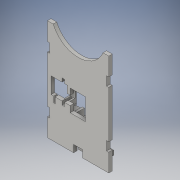
# Autodesk Inventor part: Backhalf
Saved by Autodesk Inventor 2016 (Build 200138000, 138)
## iProperties
Created: 2017-03-04
Part Number: Backhalf
Material: Generic
Document SubType Name: Modeling
Designer: Owner
Density: 1 g/cm^3
Appearance: Default
Author: Owner
Autodesk Inventor part; units mm, degrees
ref_plane "YZ Plane" through (0, 0, 0) normal (1, 0, 0) x (0, 1, 0)
ref_plane "XZ Plane" through (0, 0, 0) normal (0, 1, 0) x (-1, 0, 0)
ref_plane "XY Plane" through (0, 0, 0) normal (0, 0, 1) x (1, 0, 0)
sketch "Sketch1" plane through (0, 0, 0) normal (0, 0, 1) x (1, 0, 0)
  line L0 (31.75, -57.15) -> (31.75, 82.55)
  line L1 (31.75, 82.55) -> (-44.45, 82.55)
  line L2 (-44.45, 82.55) -> (-44.45, -57.15)
  arc A0 (-44.45, -57.15) -> (31.75, -57.15) centre (-6.35, -57.15) ccw
  line L3 (31.75, -57.15) -> (31.75, -209.55)
  line L4 (31.75, -209.55) -> (-44.45, -209.55)
  line L5 (-44.45, -209.55) -> (-44.45, -57.15)
  line L6 (31.75, -57.15) -> (-44.45, -57.15)
  circle A1 centre (-6.35, -57.15) radius 38.1
  point P0 (0, 0)
  dimension "d0" = 152.4
  dimension "d6" = 76.2
  constraints: 14 end point, 3 perpendicular, 2 centre point, 2 point on circle, 2 tangent, 1 coincident, 1 concentric, 1 vertical
  measures "d0" distance of L0.start L3.end
  measures "d6" distance of L3.end L4.end
extrude "Extrusion1" add sketch "Sketch1" against normal blind 5 contours L3 L4 L5 A0
sketch "Sketch2" plane through (0, 0, 0) normal (0, 0, 1) x (1, 0, 0)
  arc A0 (-44.45, -57.15) -> (31.75, -57.15) centre (-6.35, -57.15) ccw projected
  line L0 (31.75, -57.15) -> (31.75, -209.55) projected
  line L1 (-44.45, -57.15) -> (31.75, -57.15)
  line L2 (31.75, -57.15) -> (31.75, -72.15)
  line L3 (31.75, -72.15) -> (-44.45, -72.15)
  line L4 (-44.45, -72.15) -> (-44.45, -57.15)
  point P0 (0, 0)
  dimension "d3" = 15
  constraints: 8 end point, 2 parallel, 1 horizontal, 1 perpendicular, 1 point on line
  measures "d3" distance of L3.end L1.start
extrude "Extrusion2" cut sketch "Sketch2" against normal blind 5 contours L1 A0 L3 | A0 L3 L4 | L0 L3 A0
sketch "Sketch3" plane through (0, 0, -5) normal (0, 0, -1) x (-1, 0, 0)
  line L0 (16.51, -146.85) -> (16.51, -159.55) projected
  line L1 (-3.81, -159.55) -> (-3.81, -146.85) projected
  line L2 (16.51, -159.55) -> (16.51, -161.55)
  line L3 (-3.81, -146.85) -> (-3.81, -144.85)
  line L4 (4.857, -150.5555) -> (16.51, -161.55)
  line L5 (8.3369, -156.3105) -> (-3.81, -144.85)
  line L6 (16.51, -141.135) -> (12.446, -141.135)
  line L7 (16.51, -165.265) -> (12.446, -165.265)
  line L8 (16.51, -141.135) -> (17.51, -141.135)
  line L9 (17.51, -141.135) -> (17.51, -138.135)
  line L10 (17.51, -138.135) -> (-3.81, -138.135)
  line L11 (-3.81, -138.135) -> (-3.81, -163.265)
  line L12 (-3.81, -163.265) -> (-3.81, -164.265)
  line L13 (17.51, -138.135) -> (17.51, -165.265)
  line L14 (17.51, -165.265) -> (17.51, -168.265)
  line L15 (17.51, -168.265) -> (-3.81, -168.265)
  line L16 (-3.81, -168.265) -> (-3.81, -164.265)
  point P0 (0, 0)
  point P1 (17.51, -164.265)
  dimension "d7" = 2
  dimension "d8" = 2
  dimension "d28" = 1
  dimension "d29" = 3
  dimension "d30" = 1
  dimension "d73" = 3
  constraints: 30 end point, 5 perpendicular, 3 horizontal, 3 point on line, 3 vertical, 1 parallel, 4 other
  measures "d7" distance of L0.end L2.end
  measures "d8" distance of L1.end L3.end
  measures "d28" distance of L6.start L8.end
  measures "d29" distance of L8.end L9.end
  measures "d30" distance of L11.end L12.end
  measures "d73" distance of L13.end L14.end
extrude "Extrusion3" cut sketch "Sketch3" against normal blind 5
sketch "Sketch4" plane through (0, 0, -5) normal (0, 0, -1) x (-1, 0, 0)
  line L0 (-31.75, -72.15) -> (-28.673, -72.15) projected
  line L1 (-31.75, -72.15) -> (-36.75, -72.15)
  line L2 (-36.75, -72.15) -> (-36.75, -209.55)
  line L3 (-36.75, -209.55) -> (-36.75, -214.55)
  line L4 (-36.75, -214.55) -> (44.45, -214.55)
  line L5 (44.45, -214.55) -> (49.45, -214.55)
  line L6 (49.45, -214.55) -> (49.45, -72.15)
  line L7 (49.45, -72.15) -> (44.45, -72.15)
  line L8 (44.45, -72.15) -> (44.45, -214.55)
  line L9 (44.45, -214.55) -> (49.45, -214.55)
  line L10 (49.45, -214.55) -> (49.45, -72.15)
  line L11 (49.45, -214.55) -> (-36.75, -214.55)
  line L12 (-36.75, -214.55) -> (-36.75, -209.55)
  line L13 (-36.75, -209.55) -> (49.45, -209.55)
  line L14 (49.45, -209.55) -> (49.45, -214.55)
  line L15 (-36.75, -214.55) -> (-31.75, -214.55)
  line L16 (-31.75, -214.55) -> (-31.75, -72.15)
  line L17 (-31.75, -72.15) -> (-36.75, -72.15)
  line L18 (-36.75, -72.15) -> (-36.75, -214.55)
  point P0 (0, 0)
  dimension "d11" = 5
  dimension "d12" = 5
  dimension "d13" = 5
  constraints: 36 end point, 6 parallel, 6 perpendicular, 4 horizontal, 3 point on line
  measures "d11" distance of L0.start L1.end
  measures "d12" distance of L2.end L3.end
  measures "d13" distance of L4.end L5.end
extrude "Extrusion4" add sketch "Sketch4" against normal blind 5
sketch "Sketch6" plane through (-49.45, -214.55, 0) normal (0, -1, 0) x (1, 0, 0)
  line L0 (32.94, 0) -> (53.26, 0) projected
  line L1 (43.1, 0) -> (36.75, 0)
  line L2 (36.75, 0) -> (49.45, 0)
  line L3 (86.2, -5) -> (0, -5) projected
  line L4 (49.45, 0) -> (36.75, 0)
  line L5 (36.75, 0) -> (36.75, -5)
  line L6 (36.75, -5) -> (49.45, -5)
  line L7 (49.45, -5) -> (49.45, 0)
  point P0 (64.1616, -5)
  dimension "d18" = 6.35
  dimension "d19" = 12.7
  constraints: 12 end point, 2 parallel, 2 point on line, 1 collinear, 1 horizontal, 1 midpoint, 1 perpendicular
  measures "d18" distance of L1.start L1.end
  measures "d19" distance of L1.end L2.end
extrude "Extrusion6" add sketch "Sketch6" along normal blind 10.16
sketch "Sketch7" plane through (0, 0, -5) normal (0, 0, -1) x (-1, 0, 0)
  line L0 (12.7, -224.71) -> (0, -224.71) projected
  line L1 (6.35, -224.71) -> (6.35, -220.9)
  circle A0 centre (6.35, -220.9) radius 1.75
  point P0 (0, 0)
  dimension "d26" = 3.81
  dimension "d27" = 3.5
  constraints: 2 end point, 1 centre point, 1 coincident, 1 midpoint, 1 vertical
  measures "d26" distance of L1.start L1.end
  measures "d27" diameter of A0
extrude "Extrusion7" cut sketch "Sketch7" against normal blind 6.35
sketch "Sketch8" plane through (0, 0, -5) normal (0, 0, -1) x (-1, 0, 0)
  line L0 (44.45, -136.69) -> (28.448, -136.69) projected
  line L1 (44.45, -158.28) -> (44.45, -137.96) projected
  line L2 (44.45, -136.69) -> (44.45, -137.96) projected
  line L3 (44.45, -158.28) -> (44.45, -159.55) projected
  line L4 (44.45, -159.55) -> (28.448, -159.55) projected
  line L5 (39.116, -159.55) -> (40.132, -159.55) projected
  line L6 (39.116, -159.55) -> (39.116, -162.09) projected
  line L7 (40.132, -162.09) -> (39.116, -162.09) projected
  line L8 (40.132, -159.55) -> (40.132, -162.09) projected
  line L9 (25.908, -137.96) -> (21.59, -137.96) projected
  line L10 (21.59, -153.2) -> (21.59, -137.96) projected
  line L11 (21.59, -158.28) -> (21.59, -153.2) projected
  line L12 (25.908, -158.28) -> (21.59, -158.28) projected
  line L13 (25.908, -158.28) -> (25.908, -164.122) projected
  line L14 (25.908, -164.122) -> (28.448, -164.122) projected
  line L15 (28.448, -158.28) -> (28.448, -164.122) projected
  line L16 (44.45, -158.28) -> (28.448, -158.28) projected
  line L17 (44.45, -158.28) -> (44.45, -137.96) projected
  line L18 (44.45, -137.96) -> (28.448, -137.96) projected
  line L19 (28.448, -132.118) -> (28.448, -137.96) projected
  line L20 (25.908, -132.118) -> (28.448, -132.118) projected
  line L21 (25.908, -132.118) -> (25.908, -137.96) projected
  line L22 (25.908, -136.69) -> (21.59, -136.69) projected
  line L23 (21.59, -136.69) -> (21.59, -137.96) projected
  line L24 (25.908, -159.55) -> (21.59, -159.55) projected
  line L25 (21.59, -159.55) -> (16.51, -159.55)
  line L26 (21.59, -146.85) -> (16.51, -146.85)
  line L27 (17.51, -140.135) -> (17.51, -166.265) projected
  line L28 (44.45, -159.55) -> (21.59, -159.55)
  line L29 (21.59, -159.55) -> (21.59, -136.69)
  line L30 (21.59, -136.69) -> (44.45, -136.69)
  line L31 (44.45, -136.69) -> (44.45, -159.55)
  line L32 (28.448, -132.118) -> (25.908, -132.118)
  line L33 (25.908, -132.118) -> (25.908, -136.69)
  line L34 (25.908, -136.69) -> (28.448, -136.69)
  line L35 (28.448, -136.69) -> (28.448, -132.118)
  line L36 (25.908, -159.55) -> (28.448, -159.55)
  line L37 (28.448, -159.55) -> (28.448, -164.122)
  line L38 (28.448, -164.122) -> (25.908, -164.122)
  line L39 (25.908, -164.122) -> (25.908, -159.55)
  line L40 (40.132, -162.09) -> (39.116, -162.09)
  line L41 (39.116, -162.09) -> (39.116, -159.55)
  line L42 (39.116, -159.55) -> (40.132, -159.55)
  line L43 (40.132, -159.55) -> (40.132, -162.09)
  line L44 (16.51, -146.85) -> (21.59, -146.85)
  line L45 (21.59, -146.85) -> (21.59, -159.55)
  line L46 (21.59, -159.55) -> (16.51, -159.55)
  line L47 (16.51, -159.55) -> (16.51, -146.85)
  line L48 (40.132, -159.55) -> (40.64, -159.55)
  line L49 (40.64, -159.55) -> (40.64, -167.805)
  line L50 (40.64, -167.805) -> (39.116, -167.805)
  line L51 (39.116, -167.805) -> (38.608, -167.805)
  line L52 (38.608, -167.805) -> (38.608, -159.55)
  line L53 (40.64, -167.805) -> (38.608, -167.805)
  line L54 (38.608, -167.805) -> (38.608, -159.55)
  line L55 (38.608, -159.55) -> (40.64, -159.55)
  line L56 (40.64, -159.55) -> (40.64, -167.805)
  line L57 (28.448, -136.69) -> (28.948, -136.69)
  line L58 (28.948, -136.69) -> (28.948, -132.118)
  line L59 (28.948, -132.118) -> (28.948, -131.618)
  line L60 (28.948, -131.618) -> (25.908, -131.618)
  line L61 (25.908, -131.618) -> (25.408, -131.618)
  line L62 (25.408, -131.618) -> (25.408, -136.69)
  line L63 (44.45, -148.12) -> (42.0007, -148.12)
  line L64 (28.448, -164.122) -> (28.448, -158.28)
  line L65 (25.908, -164.122) -> (28.448, -164.122)
  line L66 (25.908, -164.122) -> (25.908, -158.28)
  line L67 (28.448, -164.122) -> (25.908, -164.122)
  line L68 (25.908, -164.122) -> (25.908, -159.55)
  line L69 (28.448, -159.55) -> (28.448, -164.122)
  line L70 (28.948, -159.55) -> (28.948, -164.122)
  line L71 (28.948, -164.122) -> (28.948, -164.622)
  line L72 (28.948, -164.622) -> (25.908, -164.622)
  line L73 (25.908, -164.622) -> (25.408, -164.622)
  line L74 (25.408, -164.622) -> (25.408, -159.55)
  line L75 (28.948, -159.55) -> (25.408, -159.55)
  line L76 (25.408, -159.55) -> (25.408, -164.622)
  line L77 (25.408, -164.622) -> (28.948, -164.622)
  line L78 (28.948, -164.622) -> (28.948, -159.55)
  point P0 (0, 0)
  dimension "d33" = 0.508
  dimension "d34" = 8.255
  dimension "d35" = 0.508
  dimension "d45" = 0.5
  dimension "d46" = 0.5
  dimension "d47" = 0.5
  constraints: 100 end point, 14 parallel, 12 perpendicular, 10 horizontal, 9 point on line, 9 symmetric about line, 1 midpoint, 1 vertical, 3 other
  measures "d33" distance of L42.end L48.end
  measures "d34" distance of L48.end L49.end
  measures "d35" distance of L50.end L51.end
  measures "d45" distance of L34.end L57.end
  measures "d46" distance of L58.end L59.end
  measures "d47" distance of L60.end L61.end
extrude "Extrusion8" cut sketch "Sketch8" against normal blind 25.4
sketch "Sketch9" plane through (0, 0, -5) normal (0, 0, -1) x (-1, 0, 0)
  line L0 (25.908, -132.118) -> (28.448, -132.118) projected
  line L1 (28.448, -132.118) -> (28.948, -132.118)
  line L2 (28.948, -132.118) -> (28.948, -131.618)
  line L3 (28.948, -131.618) -> (30.948, -131.618)
  line L4 (30.948, -131.618) -> (30.948, -136.69)
  line L5 (44.45, -136.69) -> (28.948, -136.69) projected
  line L6 (30.948, -136.69) -> (30.948, -136.19)
  line L7 (30.948, -136.19) -> (28.948, -136.19)
  line L8 (28.948, -136.19) -> (28.948, -131.618)
  line L9 (30.948, -131.618) -> (30.948, -129.618)
  line L10 (30.948, -129.618) -> (25.908, -129.618)
  line L11 (27.178, -132.118) -> (27.178, -133.3917)
  line L12 (28.448, -132.118) -> (25.908, -132.118)
  line L13 (25.908, -132.118) -> (25.408, -132.118)
  line L14 (25.408, -132.118) -> (25.408, -131.618)
  line L15 (25.408, -131.618) -> (23.408, -131.618)
  line L16 (23.408, -131.618) -> (23.408, -136.69)
  line L17 (9.906, -136.69) -> (25.908, -136.69)
  line L18 (23.408, -136.69) -> (23.408, -136.19)
  line L19 (23.408, -136.19) -> (25.408, -136.19)
  line L20 (25.408, -136.19) -> (25.408, -131.618)
  line L21 (23.408, -131.618) -> (23.408, -129.618)
  line L22 (23.408, -129.618) -> (28.448, -129.618)
  line L23 (28.948, -131.618) -> (25.408, -131.618)
  line L24 (44.45, -159.55) -> (44.45, -136.69) projected
  line L25 (44.45, -148.12) -> (41.4953, -148.12)
  line L26 (25.908, -164.122) -> (28.448, -164.122)
  line L27 (28.448, -164.122) -> (28.948, -164.122)
  line L28 (28.948, -164.122) -> (28.948, -164.622)
  line L29 (28.948, -164.622) -> (30.948, -164.622)
  line L30 (30.948, -164.622) -> (30.948, -159.55)
  line L31 (44.45, -159.55) -> (28.448, -159.55)
  line L32 (30.948, -159.55) -> (30.948, -160.05)
  line L33 (30.948, -160.05) -> (28.948, -160.05)
  line L34 (28.948, -160.05) -> (28.948, -164.622)
  line L35 (30.948, -164.622) -> (30.948, -166.622)
  line L36 (30.948, -166.622) -> (25.908, -166.622)
  line L37 (27.178, -164.122) -> (27.178, -162.8483)
  line L38 (28.448, -164.122) -> (25.908, -164.122)
  line L39 (25.908, -164.122) -> (25.408, -164.122)
  line L40 (25.408, -164.122) -> (25.408, -164.622)
  line L41 (25.408, -164.622) -> (23.408, -164.622)
  line L42 (23.408, -164.622) -> (23.408, -159.55)
  line L43 (9.906, -159.55) -> (25.908, -159.55)
  line L44 (23.408, -159.55) -> (23.408, -160.05)
  line L45 (23.408, -160.05) -> (25.408, -160.05)
  line L46 (25.408, -160.05) -> (25.408, -164.622)
  line L47 (23.408, -164.622) -> (23.408, -166.622)
  line L48 (23.408, -166.622) -> (28.448, -166.622)
  line L49 (28.948, -164.622) -> (25.408, -164.622)
  line L50 (23.408, -131.618) -> (30.948, -131.618)
  line L51 (30.948, -131.618) -> (30.948, -129.618)
  line L52 (30.948, -129.618) -> (23.408, -129.618)
  line L53 (23.408, -129.618) -> (23.408, -131.618)
  line L54 (30.948, -166.622) -> (23.408, -166.622)
  line L55 (23.408, -166.622) -> (23.408, -164.622)
  line L56 (23.408, -164.622) -> (30.948, -164.622)
  line L57 (30.948, -164.622) -> (30.948, -166.622)
  line L58 (28.948, -136.19) -> (30.948, -136.19)
  line L59 (30.948, -136.19) -> (30.948, -131.618)
  line L60 (30.948, -131.618) -> (28.948, -131.618)
  line L61 (28.948, -131.618) -> (28.948, -136.19)
  line L62 (25.408, -136.19) -> (23.408, -136.19)
  line L63 (23.408, -136.19) -> (23.408, -131.618)
  line L64 (23.408, -131.618) -> (25.408, -131.618)
  line L65 (25.408, -131.618) -> (25.408, -136.19)
  line L66 (28.948, -164.622) -> (30.948, -164.622)
  line L67 (30.948, -164.622) -> (30.948, -160.05)
  line L68 (30.948, -160.05) -> (28.948, -160.05)
  line L69 (28.948, -160.05) -> (28.948, -164.622)
  line L70 (25.408, -164.622) -> (23.408, -164.622)
  line L71 (23.408, -164.622) -> (23.408, -160.05)
  line L72 (23.408, -160.05) -> (25.408, -160.05)
  line L73 (25.408, -160.05) -> (25.408, -164.622)
  point P0 (0, 0)
  point P1 (28.448, -136.69)
  dimension "d36" = 0.5
  dimension "d37" = 0.5
  dimension "d38" = 2
  dimension "d39" = 0.5
  dimension "d40" = 2
  constraints: 142 end point, 37 symmetric about line, 12 parallel, 12 point on line, 10 horizontal, 10 perpendicular, 2 midpoint, 1 collinear, 1 vertical
  measures "d36" distance of L0.end L1.end
  measures "d37" distance of L1.end L2.end
  measures "d38" distance of L2.end L3.end
  measures "d39" distance of L4.end L6.end
  measures "d40" distance of L3.end L9.end
extrude "Extrusion9" add sketch "Sketch9" along normal blind 7.6962 contours L20 L19 L16 L15 L14 | L15 L21 L22 L10 L9 L3 L23 | L2 L3 L4 L7 L8 | L40 L41 L42 L45 L46 | L49 L29 L35 L36 L48 L47 L41 | L34 L33 L30 L29 L28
sketch "Sketch10" plane through (0, 0, -12.6962) normal (0, 0, -1) x (-1, 0, 0)
  line L0 (30.948, -129.618) -> (30.948, -136.19) projected
  line L1 (23.408, -160.05) -> (23.408, -166.622) projected
  line L2 (30.948, -129.618) -> (23.408, -129.618)
  line L3 (23.408, -129.618) -> (23.408, -166.622)
  line L4 (23.408, -166.622) -> (30.948, -166.622)
  line L5 (30.948, -166.622) -> (30.948, -129.618)
  point P0 (0, 0)
  constraints: 8 end point, 2 parallel, 1 horizontal, 1 perpendicular
extrude "Extrusion10" add sketch "Sketch10" along normal blind 2.0066
ref_plane "Work Plane1" through (-5.588, -193.548, -26.4528) normal (1, 0, 0) x (0, 0, 1)
sketch "Sketch11" plane through (-5.588, -193.548, -26.4528) normal (1, 0, 0) x (0, 0, 1)
  line L0 (6.35, -16.002) -> (6.35, -10.16) projected
  line L1 (6.35, -16.002) -> (6.35, -18.502)
  line L2 (6.35, 10.16) -> (6.35, 16.002) projected
  line L3 (6.35, 16.002) -> (6.35, 18.502)
  line L4 (21.4528, -121.398) -> (21.4528, 21.002) projected
  line L5 (6.35, -18.502) -> (21.4528, -18.502)
  line L6 (21.4528, -18.502) -> (21.4528, 18.502)
  line L7 (21.4528, 18.502) -> (6.35, 18.502)
  line L8 (6.35, 18.502) -> (6.35, -18.502)
  point P0 (26.4528, -193.548)
  dimension "d48" = 2.5
  dimension "d49" = 2.5
  constraints: 12 end point, 2 parallel, 2 vertical, 1 horizontal, 1 perpendicular, 1 point on line
  measures "d48" distance of L0.start L1.end
  measures "d49" distance of L2.end L3.end
extrude "Extrusion11" add sketch "Sketch11" against normal blind 5.04
sketch "Sketch12" plane through (-5.588, -193.548, -26.4528) normal (1, 0, 0) x (0, 0, -1)
  line L0 (-6.35, 18.502) -> (-21.4528, 18.502) projected
  line L1 (-21.4528, -18.502) -> (-21.4528, 18.502) projected
  line L2 (-21.4528, -18.502) -> (-6.35, -18.502) projected
  line L3 (-6.35, -18.502) -> (-6.35, 18.502) projected
  point P0 (-26.4528, 193.548)
extrude "Extrusion12" add sketch "Sketch12" along normal blind 10
sketch "Sketch13" plane through (-10.628, -212.05, -20.1028) normal (0, 0, -1) x (-1, 0, 0)
  line L0 (-21.042, 28.662) -> (-5.04, 28.662) projected
  line L1 (-21.042, 28.662) -> (-21.042, 8.342) projected
  line L2 (-21.042, 8.342) -> (-5.04, 8.342) projected
  line L3 (-5.04, 2.5) -> (-5.04, 8.342) projected
  line L4 (-2.5, 2.5) -> (-5.04, 2.5) projected
  line L5 (-2.5, 2.5) -> (-2.5, 8.342) projected
  line L6 (-2.5, 8.342) -> (1.818, 8.342) projected
  line L7 (1.818, 13.422) -> (1.818, 8.342) projected
  line L8 (1.818, 28.662) -> (1.818, 13.422) projected
  line L9 (-2.5, 28.662) -> (1.818, 28.662) projected
  line L10 (-2.5, 28.662) -> (-2.5, 34.504) projected
  line L11 (-2.5, 34.504) -> (-5.04, 34.504) projected
  line L12 (-5.04, 28.662) -> (-5.04, 34.504) projected
  line L13 (-2.5, 29.932) -> (1.818, 29.932) projected
  line L14 (-21.042, 29.932) -> (-5.04, 29.932) projected
  line L15 (-2.5, 7.072) -> (1.818, 7.072) projected
  line L16 (-21.042, 7.072) -> (-5.04, 7.072) projected
  line L17 (-2.5, 29.932) -> (-2, 29.932)
  line L18 (-2, 29.932) -> (-2, 30.432)
  line L19 (-2, 30.432) -> (0, 30.432)
  line L20 (0, 37.004) -> (0, 0) projected
  line L21 (-2, 30.432) -> (-2, 34.504)
  line L22 (-2, 34.504) -> (-2, 35.004)
  line L23 (-2, 35.004) -> (-5.04, 35.004)
  line L24 (-5.04, 35.004) -> (-5.54, 35.004)
  line L25 (-5.54, 35.004) -> (-5.54, 29.932)
  line L26 (-5.54, 29.932) -> (-7.54, 29.932)
  line L27 (-7.54, 29.932) -> (-7.54, 35.004)
  line L28 (-7.54, 35.004) -> (-7.54, 37.004)
  line L29 (-15.04, 37.004) -> (0, 37.004) projected
  line L30 (-7.54, 37.004) -> (0, 37.004)
  line L31 (0, 37.004) -> (0, 30.432)
  line L32 (-2, 29.932) -> (0, 29.932)
  line L33 (0, 29.932) -> (0, 37.004)
  line L34 (0, 37.004) -> (-2, 37.004)
  line L35 (-2, 37.004) -> (-2, 29.932)
  line L36 (-21.042, 18.502) -> (-17.938, 18.502)
  line L37 (-21.042, 8.342) -> (-5.04, 8.342)
  line L38 (1.818, 8.342) -> (1.818, 23.582)
  line L39 (-2.5, 8.342) -> (1.818, 8.342)
  line L40 (-2.5, 8.342) -> (-2.5, 2.5)
  line L41 (-2.5, 2.5) -> (-5.04, 2.5)
  line L42 (-5.04, 8.342) -> (-5.04, 2.5)
  line L43 (-2.5, 7.072) -> (1.818, 7.072)
  line L44 (-21.042, 7.072) -> (-5.04, 7.072)
  line L45 (-2.5, 7.072) -> (-2, 7.072)
  line L46 (-2, 7.072) -> (-2, 6.572)
  line L47 (-2, 6.572) -> (0, 6.572)
  line L48 (0, 0) -> (0, 37.004)
  line L49 (-2, 6.572) -> (-2, 2.5)
  line L50 (-2, 2.5) -> (-2, 2)
  line L51 (-2, 2) -> (-5.04, 2)
  line L52 (-5.04, 2) -> (-5.54, 2)
  line L53 (-5.54, 2) -> (-5.54, 7.072)
  line L54 (-5.54, 7.072) -> (-7.54, 7.072)
  line L55 (-7.54, 7.072) -> (-7.54, 2)
  line L56 (-7.54, 2) -> (-7.54, 0)
  line L57 (-15.04, 0) -> (0, 0)
  line L58 (-7.54, 0) -> (0, 0)
  line L59 (0, 0) -> (0, 6.572)
  line L60 (-2, 7.072) -> (0, 7.072)
  line L61 (0, 7.072) -> (0, 0)
  line L62 (0, 0) -> (-2, 0)
  line L63 (-2, 0) -> (-2, 7.072)
  point P0 (-10.628, 212.05)
  dimension "d0" = 152.4
  dimension "d19" = 12.7
  dimension "d28" = 1
  dimension "d29" = 3
  dimension "d30" = 1
  dimension "d73" = 3
  dimension "d54" = 0.5
  dimension "d55" = 0.5
  dimension "d56" = 2
  dimension "d57" = 0.5
  dimension "d58" = 0.5
  dimension "d59" = 2
  dimension "d60" = 2
  constraints: 74 end point, 17 symmetric about line, 16 point on line, 4 perpendicular, 3 parallel, 2 horizontal, 1 collinear, 1 midpoint, 1 vertical
  measures "d54" distance of L13.start L17.end
  measures "d55" distance of L17.end L18.end
  measures "d56" distance of L18.end L19.end
  measures "d57" distance of L21.end L22.end
  measures "d58" distance of L23.end L24.end
  measures "d59" distance of L25.end L26.end
  measures "d60" distance of L27.end L28.end
extrude "Extrusion13" add sketch "Sketch13" along normal blind 12 contours L14 L27 L28 L29 L35 L23 L24 L25 | L53 L52 L51 L63 L57 L56 L55 L16 | L35 L29 L20 L19 L21 L22 | L15 L20 L47 L46 | L50 L49 L47 L20 L57 L63
sketch "Sketch14" plane through (-30.948, -166.622, -5) normal (-1, 0, 0) x (0, 0, 1)
  line L0 (-9.7028, 18.744) -> (-9.7028, -2.006) projected
  line L1 (0, 94.472) -> (0, -47.928) projected
  line L2 (-9.7028, 0) -> (0, 0)
  line L3 (0, 0) -> (0, -2.006)
  line L4 (0, -2.006) -> (-9.7028, -2.006)
  line L5 (-9.7028, -2.006) -> (-9.7028, 0)
  point P0 (5, 166.622)
  constraints: 8 end point, 2 parallel, 1 horizontal, 1 perpendicular, 1 point on line
extrude "Extrusion14" add sketch "Sketch14" against normal blind 7.5438
sketch "Sketch15" plane through (0, 0, -5) normal (0, 0, -1) x (-1, 0, 0)
  line L0 (36.09, -168.628) -> (36.09, -191.4473) projected
  line L1 (36.09, -168.628) -> (36.09, -191.4473) projected
  line L2 (21.59, -168.628) -> (21.59, -191.4473) projected
  line L3 (36.09, -191.4473) -> (36.09, -186.4473)
  line L4 (36.09, -168.628) -> (36.09, -173.628)
  line L5 (36.09, -186.4473) -> (39.09, -186.4473)
  line L6 (39.09, -186.4473) -> (39.09, -173.628)
  line L7 (39.09, -173.628) -> (36.09, -173.628)
  line L8 (36.09, -173.628) -> (36.09, -186.4473)
  line L9 (21.59, -168.628) -> (21.59, -173.628)
  line L10 (21.59, -173.628) -> (18.59, -173.628)
  line L11 (18.59, -173.628) -> (18.59, -186.4473)
  line L12 (18.59, -186.4473) -> (21.59, -186.4473)
  line L13 (21.59, -186.4473) -> (21.59, -173.628)
  point P0 (0, 0)
  dimension "d65" = 5
  dimension "d66" = 5
  dimension "d67" = 3
  dimension "d68" = 3
  constraints: 22 end point, 4 parallel, 3 point on line, 2 horizontal, 2 perpendicular
  measures "d65" distance of L0.end L3.end
  measures "d66" distance of L0.start L4.end
  measures "d67" distance of L6.end L7.end
  measures "d68" distance of L9.end L10.end
extrude "Extrusion15" add sketch "Sketch15" along normal blind 16
sketch "Sketch16" plane through (-39.09, -186.4473, -5) normal (0, -1, 0) x (1, 0, 0)
  line L0 (3, -13.4528) -> (17.5, -13.4528) projected
  line L1 (0, 0) -> (0, -16) projected
  line L2 (0, -13.4528) -> (20.5, -13.4528)
  line L3 (20.5, -13.4528) -> (20.5, 0)
  line L4 (20.5, 0) -> (0, 0)
  line L5 (0, 0) -> (0, -13.4528)
  point P0 (39.09, 5)
  constraints: 8 end point, 2 parallel, 1 horizontal, 1 perpendicular, 1 point on line
extrude "Extrusion16" add sketch "Sketch16" against normal blind 12.819
sketch "Sketch17" plane through (0, 0, -5) normal (0, 0, -1) x (-1, 0, 0)
  line L0 (-7.25, -200.427) -> (-26.75, -200.427) projected
  line L1 (-26.75, -200.427) -> (-26.75, -202.177) projected
  line L2 (-7.25, -202.177) -> (-26.75, -202.177) projected
  line L3 (-7.25, -200.427) -> (-7.25, -202.177) projected
  line L4 (-7.25, -200.427) -> (-11.25, -200.427)
  line L5 (-11.25, -200.427) -> (-11.25, -200.177)
  line L6 (-11.25, -200.177) -> (-11.25, -198.177)
  line L7 (-11.25, -198.177) -> (-7.25, -198.177)
  line L8 (-7.25, -198.177) -> (-5.25, -198.177)
  line L9 (-11.25, -200.177) -> (-7.25, -200.177)
  line L10 (-7.25, -200.177) -> (-7, -200.177)
  line L11 (-7, -200.177) -> (-7, -202.177)
  line L12 (-7, -202.177) -> (-7, -202.427)
  line L13 (-7, -202.427) -> (-11.25, -202.427)
  line L14 (-11.25, -202.427) -> (-11.25, -204.427)
  line L15 (-11.25, -204.427) -> (-5.25, -204.427)
  line L16 (-5.25, -204.427) -> (-5.25, -198.177)
  line L17 (-17, -202.177) -> (-17, -205.7109)
  line L18 (-26.75, -200.427) -> (-7.25, -200.427)
  line L19 (-26.75, -202.177) -> (-7.25, -202.177)
  line L20 (-26.75, -200.427) -> (-26.75, -202.177)
  line L21 (-26.75, -200.427) -> (-22.75, -200.427)
  line L22 (-22.75, -200.427) -> (-22.75, -200.177)
  line L23 (-22.75, -200.177) -> (-22.75, -198.177)
  line L24 (-22.75, -198.177) -> (-26.75, -198.177)
  line L25 (-26.75, -198.177) -> (-28.75, -198.177)
  line L26 (-22.75, -200.177) -> (-26.75, -200.177)
  line L27 (-26.75, -200.177) -> (-27, -200.177)
  line L28 (-27, -200.177) -> (-27, -202.177)
  line L29 (-27, -202.177) -> (-27, -202.427)
  line L30 (-27, -202.427) -> (-22.75, -202.427)
  line L31 (-22.75, -202.427) -> (-22.75, -204.427)
  line L32 (-22.75, -204.427) -> (-28.75, -204.427)
  line L33 (-28.75, -204.427) -> (-28.75, -198.177)
  point P0 (0, 0)
  dimension "d74" = 4
  dimension "d75" = 0.25
  dimension "d76" = 2
  dimension "d77" = 2
  dimension "d78" = 0.25
  dimension "d79" = 0.25
  dimension "d80" = 2
  constraints: 54 end point, 16 symmetric about line, 12 point on line, 6 perpendicular, 2 vertical, 1 horizontal, 1 midpoint
  measures "d74" distance of L0.start L4.end
  measures "d75" distance of L4.end L5.end
  measures "d76" distance of L5.end L6.end
  measures "d77" distance of L7.end L8.end
  measures "d78" distance of L9.end L10.end
  measures "d79" distance of L11.end L12.end
  measures "d80" distance of L13.end L14.end
extrude "Extrusion17" add sketch "Sketch17" along normal blind 10 contours L6 L7 L8 L16 L15 L14 L13 L12 L11 L10 L9 | L26 L27 L28 L29 L30 L31 L32 L33 L25 L24 L23
sketch "Sketch18" plane through (0, 0, -5) normal (0, 0, -1) x (-1, 0, 0)
  line L0 (-36.75, -72.15) -> (-28.673, -72.15) projected
  line L1 (-36.75, -72.15) -> (-36.75, -97.55)
  line L2 (-36.75, -214.55) -> (-36.75, -72.15) projected
  line L3 (-36.75, -97.55) -> (-33.7528, -97.55)
  line L4 (-33.7528, -97.55) -> (-33.7528, -110.25)
  line L5 (-33.7528, -110.25) -> (-36.75, -110.25)
  line L6 (-36.75, -110.25) -> (-36.75, -97.55)
  line L7 (-36.75, -214.55) -> (-36.75, -189.15)
  line L8 (-36.75, -189.15) -> (-33.7528, -189.15)
  line L9 (-33.7528, -189.15) -> (-33.7528, -176.45)
  line L10 (-33.7528, -176.45) -> (-36.75, -176.45)
  line L11 (-36.75, -176.45) -> (-36.75, -189.15)
  line L12 (0, -224.71) -> (12.7, -224.71) projected
  line L13 (6.35, -224.71) -> (6.35, -239.7955)
  line L14 (49.45, -72.15) -> (41.373, -72.15)
  line L15 (49.45, -72.15) -> (49.45, -97.55)
  line L16 (49.45, -214.55) -> (49.45, -72.15)
  line L17 (49.45, -97.55) -> (46.4528, -97.55)
  line L18 (46.4528, -97.55) -> (46.4528, -110.25)
  line L19 (46.4528, -110.25) -> (49.45, -110.25)
  line L20 (49.45, -110.25) -> (49.45, -97.55)
  line L21 (49.45, -214.55) -> (49.45, -189.15)
  line L22 (49.45, -189.15) -> (46.4528, -189.15)
  line L23 (46.4528, -189.15) -> (46.4528, -176.45)
  line L24 (46.4528, -176.45) -> (49.45, -176.45)
  line L25 (49.45, -176.45) -> (49.45, -189.15)
  point P0 (0, 0)
  dimension "d83" = 25.4
  dimension "d84" = 12.7
  dimension "d85" = 2.9972
  dimension "d86" = 25.4
  dimension "d87" = 12.7
  dimension "d88" = 2.9972
  constraints: 46 end point, 11 symmetric about line, 4 parallel, 4 point on line, 2 horizontal, 2 perpendicular, 1 midpoint, 1 vertical
  measures "d83" distance of L0.start L1.end
  measures "d84" distance of L3.end L4.end
  measures "d85" distance of L4.end L5.end
  measures "d86" distance of L2.start L7.end
  measures "d87" distance of L8.end L9.end
  measures "d88" distance of L7.end L8.end
extrude "Extrusion18" cut sketch "Sketch18" against normal blind 10
sketch "Sketch20" plane through (-49.45, -224.71, 0) normal (0, -1, 0) x (1, 0, 0)
  line L0 (36.75, -5) -> (36.75, 0) projected
  line L1 (36.75, -5) -> (49.45, -5)
  line L2 (49.45, -5) -> (49.45, 0)
  line L3 (49.45, 0) -> (36.75, 0)
  line L4 (36.75, 0) -> (36.75, -5)
  constraints: 8 end point, 2 parallel, 1 horizontal, 1 perpendicular
extrude "Extrusion19" cut sketch "Sketch20" against normal blind 20.8946
body "Solid1"
